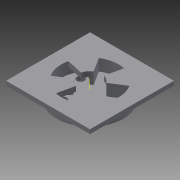
# Autodesk Inventor part: female 4 bay con
Saved by Autodesk Inventor 2015 (Build 190159000, 159)
## iProperties
Created: 2014-11-16
Part Number: female 4 bay con
Material: Generic
Document SubType Name: Modeling
Designer: ericd_000
Density: 1 g/cm^3
Appearance: Default
Author: ericd_000
Autodesk Inventor part; units mm, degrees
ref_plane "YZ Plane" through (0, 0, 0) normal (1, 0, 0) x (0, 1, 0)
ref_plane "XZ Plane" through (0, 0, 0) normal (0, 1, 0) x (-1, 0, 0)
ref_plane "XY Plane" through (0, 0, 0) normal (0, 0, 1) x (1, 0, 0)
sketch "Sketch5" plane through (0, 0, 0) normal (0, 0, 1) x (1, 0, 0)
  circle A0 centre (0, 0) radius 34
  dimension "d9" = 68
  constraints: 1 centre point, 1 coincident
  measures "d9" diameter of A0
extrude "Extrusion4" add sketch "Sketch5" along normal blind 5
sketch "Sketch6" plane through (0, 0, 5) normal (0, 0, 1) x (1, 0, 0)
  line L0 (0, 0) -> (-25.0441, 22.9955) construction
  circle A0 centre (0, 0) radius 34 construction
  line L1 (0, 0) -> (-18.239, 28.6939) construction
  line L2 (-25.0441, 22.9955) -> (-10.3123, 9.4687)
  line L3 (-18.239, 28.6939) -> (-7.5102, 11.8151)
  arc A1 (-7.5102, 11.8151) -> (-10.3123, 9.4687) centre (0, 0) ccw
  arc A2 (-18.239, 28.6939) -> (-25.0441, 22.9955) centre (0, 0) ccw
  dimension "d12" = 15
  dimension "d14" = 20
  constraints: 8 end point, 6 point on circle, 2 centre point, 2 concentric, 2 point on line
  measures "d12" angle of L0 L1
  measures "d14" distance of L0.end L2.end
extrude "Extrusion5" add sketch "Sketch6" along normal blind 14
sketch "Sketch7" plane through (-10.3123, 9.4687, 5) normal (-0.6763389, -0.7365906, 0) x (0.7365906, -0.6763389, 0)
  line L0 (-20, 14) -> (0, 14)
  line L1 (0, 14) -> (0, 8)
  line L2 (0, 8) -> (-20, 8)
  line L3 (-20, 8) -> (-20, 14)
  line L4 (14, -8.8) -> (14, 17.8) projected
  point P0 (14, -5)
  dimension "d17" = 6
  dimension "d18" = 20
  constraints: 8 end point, 2 parallel, 1 horizontal, 1 perpendicular
  measures "d17" distance between parallel lines of L0 L2
  measures "d18" distance of L0.start L0.end
revolve "Revolution1" add sketch "Sketch7" angle 30 about axis through (0, 0, 5) along (0, 0, 1)
sketch "Sketch8" plane through (0, 0, 5) normal (0, 0, 1) x (1, 0, 0)
  circle A0 centre (-21.5775, 10.5076) radius 4.5
  circle A1 centre (0, 0) radius 24 construction
  dimension "d25" = 48
  dimension "d21" = 9
  constraints: 1 centre point, 1 coincident, 3 other
  measures "d21" diameter of A0
extrude "Extrusion6" cut sketch "Sketch8" against normal up to surface (5 mm away)
pattern_circular "Circular Pattern1" count 4 over 360 about axis through (0, 0, 5) along (0, 0, 1) of "Extrusion6", "Revolution1", "Extrusion5"
sketch "Sketch9" plane through (0, 0, 0) normal (0, 0, -1) x (-1, 0, 0)
  circle A0 centre (0, 0) radius 34
  circle A1 centre (0, 0) radius 40
  dimension "d31" = 68
  dimension "d32" = 6
  constraints: 2 centre point, 2 coincident
  measures "d31" diameter of A0
  measures "d32" radial gap between concentric circles of A1 A0
extrude "Extrusion7" add sketch "Sketch9" against normal blind 19
sketch "Sketch10" plane through (0, 0, 19) normal (0, 0, 1) x (1, 0, 0)
  circle A0 centre (0, 0) radius 40
  line L0 (-50, 50) -> (50, 50)
  line L1 (50, 50) -> (50, -50)
  line L2 (50, -50) -> (-50, -50)
  line L3 (-50, -50) -> (-50, 50)
  point P0 (-50, 0)
  point P1 (0, 50)
  dimension "d35" = 100
  dimension "d36" = 100
  dimension "d37" = 80
  constraints: 8 end point, 2 midpoint, 2 parallel, 1 centre point, 1 coincident, 1 horizontal, 1 horizontal alignment, 1 perpendicular, 1 vertical alignment
  measures "d35" distance of L0.start L0.end
  measures "d36" distance of L2.end L0.start
  measures "d37" diameter of A0
extrude "Extrusion8" add sketch "Sketch10" against normal blind 5
body "Solid2"
